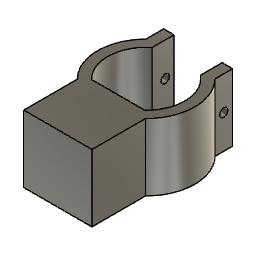
Motor Mount v1 (Autodesk Fusion 360 design; units mm, degrees)
Autodesk Fusion 360 part; units mm, degrees
note: some values were not read from the file. Set by a fixed rule: which sketch regions a step uses.
sketch "Sketch1" plane through (0, 0, 0) normal (0, 0, 1) x (1, 0, 0)
  arc A0 (7.9217, -8.3364) -> (7.9217, 8.3364) centre (0, 0) ccw
  line L0 (-7.1925, 15.5) -> (-10.2923, 15.5)
  line L1 (7.9217, -8.3364) -> (-7.9217, -8.3364)
  line L2 (7.1667, 15.5) -> (7.1667, 8.9938)
  line L3 (-10.2923, 15.5) -> (-10.2923, 10.2136)
  line L4 (10.2923, 15.5) -> (7.1667, 15.5)
  line L5 (7.9217, -8.3364) -> (-7.9217, -8.3364)
  line L6 (-10.2923, 15.5) -> (-10.2923, 10.2136)
  arc A1 (-10.2923, 10.2136) -> (-10.169, -10.3364) centre (0, 0) ccw
  line L7 (-7.1925, 15.5) -> (-7.1925, 8.9732)
  line L8 (10.2923, 10.2136) -> (10.2923, 15.5)
  arc A2 (-7.9217, 8.3364) -> (-7.9217, -8.3364) centre (0, 0) ccw
  circle A3 centre (0, 0) radius 11.5
  line L9 (-7.1925, 15.5) -> (-10.2923, 15.5)
  line L10 (10.2923, 10.2136) -> (10.2923, 15.5)
  line L11 (10.2923, 15.5) -> (7.1667, 15.5)
  arc A4 (10.169, -10.3364) -> (10.2923, 10.2136) centre (0, 0) ccw
  line L12 (10.169, -10.3364) -> (10.169, -26.3364)
  line L13 (-10.169, -10.3364) -> (-10.169, -26.3364)
  line L14 (-10.169, -26.3364) -> (10.169, -26.3364)
  dimension "d1" = 16
  dimension "d2" = 16
  constraint coincident L8.start L10.start
  constraint coincident L4.start L8.end
  constraint coincident L2.start L4.end
  constraint perpendicular L2 L4
  constraint coincident L0.start L7.start
  constraint coincident L0.end L3.start
  constraint coincident L3.end L6.end
  constraint perpendicular L0 L7
  constraint coincident A0.start L1.start
  constraint coincident L1.end L5.end
  constraint concentric A2 A3
  constraint coincident L2.end A3
  constraint vertical L2
  constraint coincident L7.end A3
  constraint vertical L7
  constraint vertical L12
  constraint vertical L13
  constraint perpendicular L12 L14
  measures "d1" distance of A4.start L12.end
  measures "d2" distance of A1.end L13.end
extrude "Extrude1" add sketch "Sketch1" along normal blind 20 contours L1 L5 A3 | A0 L0 L2 L3 L4 L6 A1 L7 L8 A2 A3 L9 L10 L11 A4 L12 L13 L14
sketch "Sketch2" plane through (10.2923, 0, 0) normal (1, 0, 0) x (0, 1, 0)
  line L0 (10.2136, 0) -> (15.5, 0)
  line L1 (15.5, 0) -> (15.5, 20)
  line L2 (15.5, 20) -> (10.2136, 20)
  line L3 (10.2136, 20) -> (10.2136, 0)
  line L4 (10.2136, 20) -> (15.5, 0) construction
  line L5 (10.2136, 0) -> (15.5, 20) construction
  circle A0 centre (12.8568, 10) radius 1.25
  dimension "d5" = 2.5
  constraint coincident L2.end L3.start
  constraint coincident L0.end L1.start
  constraint coincident L0.start L3.end
  constraint coincident L1.end L2.start
  constraint midpoint L5 A0.centre
  measures "d5" diameter of A0
extrude "Extrude2" cut sketch "Sketch2" against normal blind 21 contours A0
